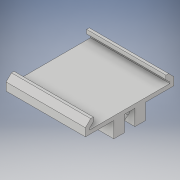
# Autodesk Inventor part: TopToBatteryJoint
Saved by Autodesk Inventor 2017 (Build 210142000, 142)
## iProperties
Created: 2020-08-23
Part Number: TopToBatteryJoint
Material: Generic
Document SubType Name: Modeling
Designer: agustin
Density: 1 g/cm^3
Appearance: Default
Author: agustin
## iProperties of the stored document battery-holder-robot_3DPrint.ipt
Created: 2021-01-25
Part Number: battery-holder-robot_3DPrint
Material: Generic
Document SubType Name: Modeling
Designer: agustin
Density: 1 g/cm^3
Appearance: Default
Author: agustin
Autodesk Inventor part; units mm, degrees
ref_plane "YZ Plane" through (0, 0, 0) normal (1, 0, 0) x (0, 1, 0)
ref_plane "XZ Plane" through (0, 0, 0) normal (0, 1, 0) x (-1, 0, 0)
sketch "Sketch1" plane through (0, 0, 0) normal (0, 0, 1) x (1, 0, 0)
  circle A0 centre (23.8656, 17.2) radius 3 projected
  line L0 (34.8656, 12.9938) -> (34.8656, 22.2) projected
  line L1 (165.9417, 25.2) -> (-24.8583, 25.2) projected
  line L2 (34.8656, 25.2) -> (-24.8606, 25.2)
  line L3 (-24.8606, 25.2) -> (-24.8606, 10.2)
  line L4 (-24.8606, 10.2) -> (34.8656, 10.2)
  line L5 (34.8656, 10.2) -> (34.8656, 25.2)
  point P0 (0, 0)
  dimension "d0" = 15
  constraints: 8 end point, 2 parallel, 2 point on line, 1 horizontal, 1 perpendicular
  measures "d0" distance of L3.end L2.end
extrude "Extrusion1" add sketch "Sketch1" along normal blind 4
sketch "Sketch2" plane through (0, 0, 4) normal (0, 0, 1) x (1, 0, 0)
  circle A0 centre (23.8656, 17.2) radius 3 projected
  line L0 (17.8656, 17.2) -> (20.8656, 22.3962)
  line L1 (20.8656, 22.3962) -> (26.8656, 22.3962)
  line L2 (26.8656, 22.3962) -> (29.8656, 17.2)
  line L3 (29.8656, 17.2) -> (26.8656, 12.0038)
  line L4 (26.8656, 12.0038) -> (20.8656, 12.0038)
  line L5 (20.8656, 12.0038) -> (17.8656, 17.2)
  circle A1 centre (23.8656, 17.2) radius 3 projected
  line L6 (34.8656, 25.2) -> (-24.8606, 25.2) projected
  line L7 (-24.8606, 25.2) -> (-24.8606, 10.2) projected
  line L8 (-24.8606, 10.2) -> (34.8656, 10.2) projected
  line L9 (34.8656, 10.2) -> (34.8656, 25.2) projected
  point P0 (0, 0)
  constraints: 12 end point, 1 coincident, 13 other
extrude "Extrusion2" add sketch "Sketch2" along normal blind 4 contours L9 L8 L7 L6
sketch "Sketch4" plane through (34.8656, 10.2, 8) normal (1, 0, 0) x (0, 0, -1)
  line L0 (8, 0.0155) -> (-4, 0.0155)
  point P0 (8, -10.2)
  dimension "d8" = 12
  constraints: 2 end point, 1 horizontal
  measures "d8" distance of L0.start L0.end
sketch "Sketch6" plane through (0, 0, 4) normal (0, 0, 1) x (1, 0, 0)
  line L0 (20.8656, 22.3962) -> (17.8656, 17.2) projected
  line L1 (17.8656, 17.2) -> (20.8656, 12.0038) projected
  line L2 (20.8656, 12.0038) -> (26.8656, 12.0038) projected
  line L3 (26.8656, 12.0038) -> (29.8656, 17.2) projected
  line L4 (29.8656, 17.2) -> (26.8656, 22.3962) projected
  circle A0 centre (23.8656, 17.2) radius 3 projected
  line L5 (26.8656, 22.3962) -> (20.8656, 22.3962) projected
  point P0 (0, 0)
extrude "Extrusion4" cut sketch "Sketch6" along normal blind 16
sketch "Sketch7" plane through (0, 0, 4) normal (0, 0, 1) x (1, 0, 0)
  circle A0 centre (23.8656, 17.2) radius 3 projected
  line L0 (17.8656, 17.2) -> (20.8656, 12.0038) projected
  line L1 (17.8656, 17.2) -> (20.8656, 22.3962)
  line L2 (20.8656, 22.3962) -> (26.8656, 22.3962)
  line L3 (26.8656, 22.3962) -> (29.8656, 17.2)
  line L4 (29.8656, 17.2) -> (26.8656, 12.0038)
  line L5 (26.8656, 12.0038) -> (20.8656, 12.0038)
  line L6 (20.8656, 12.0038) -> (17.8656, 17.2)
  point P0 (0, 0)
  constraints: 12 end point, 1 coincident, 13 other
extrude "Extrusion5" cut sketch "Sketch7" along normal blind 16
sketch "Sketch8" plane through (34.8656, 10.2, 0) normal (1, 0, 0) x (0, 0, -1)
  line L0 (-41.5, 15) -> (17.4652, 15) projected
  line L1 (17.4652, 16) -> (17.4652, 15) construction
  line L2 (15.4652, 18) -> (17.4652, 16) construction
  line L3 (14.5, 18) -> (15.4652, 18) construction
  line L4 (14.5, 18) -> (14.5, 63) construction
  arc A0 (14.5, 63) -> (12.5, 65) centre (12.5, 63) ccw construction
  line L5 (12.5, 65) -> (7.5, 65) construction
  line L6 (7.5, 65) -> (10.5, 62) construction
  line L7 (10.5, 62) -> (10.5, 20) construction
  arc A1 (8.5, 18) -> (10.5, 20) centre (8.5, 20) ccw construction
  line L8 (8.5, 18) -> (-32.5, 18) construction
  arc A2 (-34.5, 20) -> (-32.5, 18) centre (-32.5, 20) ccw construction
  line L9 (-34.5, 20) -> (-34.5, 62) construction
  line L10 (-34.5, 62) -> (-31.5, 65) construction
  line L11 (-31.5, 65) -> (-36.5, 65) construction
  arc A3 (-36.5, 65) -> (-38.5, 63) centre (-36.5, 63) ccw construction
  line L12 (-38.5, 63) -> (-38.5, 18) construction
  line L13 (-38.5, 18) -> (-39.5, 18) construction
  line L14 (-39.5, 18) -> (-41.5, 16) construction
  line L15 (-41.5, 16) -> (-41.5, 15) construction
  line L16 (0, 15) -> (17.4652, 15)
  line L17 (17.4652, 15) -> (18.4652, 15)
  line L18 (18.4652, 15) -> (18.4652, 16)
  line L19 (18.4652, 16) -> (15.4652, 19)
  line L20 (21.4652, 15) -> (21.4652, 18)
  line L21 (17.4652, 22) -> (15.4652, 22)
  line L22 (21.4652, 15) -> (21.4652, 12.0348)
  line L23 (21.4652, 12.0348) -> (0, 12.0348)
  line L24 (21.4652, 18) -> (17.4652, 22)
  line L25 (0, 0) -> (0, 15) construction
  line L26 (-32.6881, 12) -> (-32.6881, -32.4) projected
  line L27 (0, 12.0348) -> (-12, 12.0348)
  line L28 (-12, 15) -> (0, 15)
  arc A4 (-34.5, 20) -> (-32.5, 18) centre (-32.5, 20) ccw construction
  line L29 (-24, 15) -> (-41.4652, 15)
  line L30 (-41.4652, 15) -> (-42.4652, 15)
  line L31 (-42.4652, 15) -> (-42.4652, 16)
  line L32 (-42.4652, 16) -> (-39.4652, 19)
  line L33 (-45.4652, 15) -> (-45.4652, 18)
  line L34 (-41.4652, 22) -> (-39.4652, 22)
  line L35 (-45.4652, 15) -> (-45.4652, 12.0348)
  line L36 (-45.4652, 12.0348) -> (-24, 12.0348)
  line L37 (-45.4652, 18) -> (-41.4652, 22)
  line L38 (-24, 12.0348) -> (-12, 12.0348)
  line L39 (-12, 15) -> (-24, 15)
  line L40 (18.4652, 15) -> (-42.4652, 15)
  line L41 (21.4652, 12.0348) -> (-45.4652, 12.0348)
  line L42 (-45.4652, 12.0348) -> (-45.4652, 18)
  line L43 (-45.4652, 18) -> (-41.4652, 22)
  line L44 (-41.4652, 22) -> (-39.4652, 22)
  line L45 (-39.4652, 19) -> (-42.4652, 16)
  line L46 (-42.4652, 16) -> (-42.4652, 15)
  line L47 (-42.4652, 15) -> (18.4652, 15)
  line L48 (15.4652, 19) -> (15.4652, 22)
  line L49 (-39.4652, 19) -> (-39.4652, 22)
  point P0 (0, -10.2)
  point P1 (21.4652, 22)
  point P2 (-45.4652, 22)
  dimension "d16" = 3
  dimension "d17" = 4
  dimension "d18" = 4
  constraints: 64 end point, 10 perpendicular, 6 point on line, 3 equal length, 3 horizontal, 1 vertical
  measures "d16" distance of L17.end L20.start
  measures "d17" distance of L20.end point (21.465, 22)
  measures "d18" distance of L21.start point (21.465, 22)
extrude "Extrusion6" add sketch "Sketch8" against normal blind 60
sketch "Sketch9" plane through (34.8656, 22.2348, 8) normal (0, -1, 0) x (1, 0, 0)
  line L0 (0, -8) -> (0, -29.4652) projected
  line L1 (-60, -29.4652) -> (-60, 37.4652) projected
  line L2 (0, -8) -> (-60, -8)
  line L3 (-60, -8) -> (-60, 16)
  line L4 (-60, 16) -> (0, 16)
  line L5 (0, 16) -> (0, -8)
  line L6 (-60, 4) -> (0, 4)
  point P0 (-34.8656, -8)
  dimension "d21" = 24
  constraints: 10 end point, 2 midpoint, 2 parallel, 1 horizontal, 1 perpendicular, 1 point on line
  measures "d21" distance of L2.end L3.end
ref_plane "Work Plane3" through (-25.1344, 22.2348, 12) normal (0, 0, -1) x (1, 0, 0)
mirror "Mirror2" about plane through (-25.1344, 22.2348, 12) normal (0, 0, -1) of "Extrusion1", "Extrusion2"
sketch "Sketch11" plane through (26.9587, 22.2348, 20) normal (0, 0, -1) x (-1, 0, 0)
  circle A0 centre (3.0931, -5.0348) radius 3 projected
  circle A1 centre (3.0931, -5.0348) radius 7
  circle A2 centre (3.0931, -5.0348) radius 3 projected
  line L0 (-3.9069, -5.0348) -> (-0.4069, 1.0273)
  line L1 (-0.4069, 1.0273) -> (6.5931, 1.0273)
  line L2 (6.5931, 1.0273) -> (10.0931, -5.0348)
  line L3 (10.0931, -5.0348) -> (6.5931, -11.097)
  line L4 (6.5931, -11.097) -> (-0.4069, -11.097)
  line L5 (-0.4069, -11.097) -> (-3.9069, -5.0348)
  point P0 (26.9587, -22.2348)
  dimension "d25" = 14
  constraints: 12 end point, 2 coincident, 1 horizontal alignment, 15 other
extrude "Extrusion8" cut sketch "Sketch11" along normal blind 16 contours L3 L4 L5 L0 L1 L2
scale "Scale1" factors (0.5, 0.5, 0.5) then translate (2.4328, 12.6, 6) bodies 1
equation "\"d18\" = d17"
body "Solid1"
